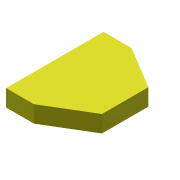
# Autodesk Inventor part: 30_Cube_Z_Focus_Drylin_NEMA_slide_part1
Saved by Autodesk Inventor 2022 (Build 260153000, 153)
## iProperties
Created: 2021-05-05
Part Number: 30_Cube_Z_Focus_Drylin_NEMA_slide_part1
Material: Generic
Document SubType Name: Modeling
Designer: diederichbenedict
Density: 1 g/cm^3
Appearance: Smooth - Yellow
Author: diederichbenedict
Autodesk Inventor part; units mm, degrees
ref_plane "YZ Plane" through (0, 0, 0) normal (1, 0, 0) x (0, 1, 0)
ref_plane "XZ Plane" through (0, 0, 0) normal (0, 1, 0) x (-1, 0, 0)
ref_plane "XY Plane" through (0, 0, 0) normal (0, 0, 1) x (1, 0, 0)
sketch "Sketch1" plane through (0, 0, 0) normal (0, 1, 0) x (-1, 0, 0)
  line L0 (-13, -11.9282) -> (10, -11.9282)
  line L1 (10, -11.9282) -> (10, 11.9282)
  line L2 (10, 11.9282) -> (-13, 11.9282)
  line L3 (-13, 11.9282) -> (-13, -11.9282)
  circle A0 centre (-8, 0) radius 4
  circle A1 centre (4, -6.9282) radius 4
  circle A2 centre (4, 6.9282) radius 4
  circle A3 centre (0, 0) radius 8 construction
  circle A4 centre (0, 0) radius 1.75
  dimension "d11" = 16
  dimension "d2" = 8
  dimension "d6" = 360
  dimension "d8" = 6
  dimension "d9" = 5
  dimension "d12" = 5
  dimension "d13" = 5
  dimension "d35" = 3.5
  constraints: 8 end point, 4 centre point, 3 coincident, 2 parallel, 1 horizontal, 1 horizontal alignment, 1 perpendicular, 9 other
  measures "d2" diameter of A0
  measures "d8" distance from line of A2.centre L1
  measures "d9" distance from line of L3 A0.centre
  measures "d12" distance from line of L2 A2.centre
  measures "d13" distance from line of L0 A1.centre
  measures "d35" diameter of A4
extrude "Extrusion1" add sketch "Sketch1" along normal blind 3
sketch "Sketch2" plane through (0, 3, 0) normal (0, 1, 0) x (1, 0, 0)
  circle A0 centre (-4, -6.9282) radius 4 projected
  circle A1 centre (-4, 6.9282) radius 4 projected
  circle A2 centre (8, 0) radius 4 projected
  line L0 (13, 11.9282) -> (-10, 11.9282) projected
  line L1 (-10, 11.9282) -> (-10, -11.9282) projected
  line L2 (-10, -11.9282) -> (13, -11.9282) projected
  line L3 (13, -11.9282) -> (13, 11.9282) projected
  circle A3 centre (0, 0) radius 1.75
  dimension "d16" = 3.5
  constraints: 1 centre point, 1 coincident
  measures "d16" diameter of A3
extrude "Extrusion2" add sketch "Sketch2" along normal blind 1.5 contours A0 | A1 | A2 | L3 L2 L1 L0
sketch "Sketch3" plane through (0, 0, 0) normal (0, -1, 0) x (1, 0, 0)
  circle A0 centre (-4, 6.9282) radius 4 projected
  circle A1 centre (-4, -6.9282) radius 4 projected
  circle A2 centre (8, 0) radius 4 projected
  line L0 (13, -11.9282) -> (-10, -11.9282) projected
  line L1 (13, 11.9282) -> (13, -11.9282) projected
  line L2 (-10, 11.9282) -> (13, 11.9282) projected
  line L3 (-10, -11.9282) -> (-10, 11.9282) construction
  line L4 (-2, 11.9282) -> (13, 2.9282)
  line L5 (13, 11.9282) -> (13, -11.9282) projected
  line L6 (13, -2.9282) -> (-2, -11.9282)
  point P0 (0, 0)
  dimension "d19" = 9
  dimension "d20" = 9
  dimension "d21" = 15
  dimension "d22" = 15
  constraints: 4 end point, 4 point on line
  measures "d19" distance from line of L2 L4.end
  measures "d20" distance from line of L0 L6.start
  measures "d21" distance from line of L6.end L1
  measures "d22" distance from line of L1 L4.start
extrude "Extrusion3" cut sketch "Sketch3" against normal through all contours L4 L2 L1 | L0 L6 L1
sketch "Sketch5" plane through (0, 0, 0) normal (0, -1, 0) x (1, 0, 0)
  line L0 (13, 2.9282) -> (-2, 11.9282) projected
  line L1 (-10, 11.9282) -> (-2, 11.9282) projected
  line L2 (-10, -11.9282) -> (-10, 11.9282) projected
  line L3 (-2, -11.9282) -> (-10, -11.9282) projected
  line L4 (-2, -11.9282) -> (13, -2.9282) projected
  line L5 (13, 2.9282) -> (13, -2.9282) projected
  circle A0 centre (-4, 6.9282) radius 4 projected
  circle A1 centre (-4, -6.9282) radius 4 projected
  circle A2 centre (8, 0) radius 4 projected
  line L6 (17, -5.193) -> (-0.8921, -15.9282)
  line L7 (-0.8921, -15.9282) -> (-14, -15.9282)
  line L8 (-14, -15.9282) -> (-14, 15.9282)
  line L9 (-14, 15.9282) -> (-0.8921, 15.9282)
  line L10 (-0.8921, 15.9282) -> (17, 5.193)
  line L11 (17, 5.193) -> (17, -5.193)
  line L12 (13, -2.9282) -> (13, -7.593)
  line L13 (13, 2.8448) -> (13, 7.593)
  line L14 (-2, -11.9282) -> (-10, -11.9282) projected
  line L15 (-10, -11.9282) -> (-10, -15.9282)
  line L16 (-10, 11.9282) -> (-2, 11.9282) projected
  line L17 (-10, 11.9282) -> (-10, 15.9282)
  line L18 (-2, -11.9282) -> (13, -2.9282) projected
  line L19 (13, -2.9282) -> (-2, -11.9282)
  line L20 (-2, -11.9282) -> (-10, -11.9282)
  line L21 (-10, -11.9282) -> (-10, 11.9282) projected
  line L22 (-10, 11.9282) -> (-2, 11.9282)
  line L23 (13, 2.9282) -> (-2, 11.9282) projected
  line L24 (13, 2.9282) -> (-2, 11.9282)
  line L25 (13, -2.9282) -> (13, 2.8448)
  point P0 (0, 0)
  dimension "d27" = 4
  constraints: 30 end point, 6 point on line, 4 collinear, 2 perpendicular, 2 vertical, 5 other
  measures "d27" distance between parallel lines of L4 L6
extrude "Extrusion5" add sketch "Sketch5" against normal up to surface (4.5 mm away) contours L0 L1 L17 L9 L10 L13 | L12 L6 L7 L15 L3 L4
sketch "Sketch6" plane through (0, 4.5, 0) normal (0, 1, 0) x (1, 0, 0)
  line L0 (13, -7.593) -> (13, 7.593) projected
  line L1 (-0.8921, 15.9282) -> (13, 7.593) projected
  line L2 (-10, 15.9282) -> (-0.8921, 15.9282) projected
  line L3 (-10, -15.9282) -> (-10, 15.9282) projected
  line L4 (-0.8921, -15.9282) -> (-10, -15.9282) projected
  line L5 (13, -7.593) -> (-0.8921, -15.9282) projected
  line L6 (13, 7.593) -> (-0.8921, 15.9282)
  line L7 (-0.8921, 15.9282) -> (-2.4356, 13.3557)
  line L8 (-2.4356, 13.3557) -> (11.4565, 5.0205)
  line L9 (11.4565, 5.0205) -> (13, 7.593)
  line L10 (13, -7.593) -> (13, 7.593) projected
  line L11 (13, -7.593) -> (-0.8921, -15.9282)
  line L12 (-0.8921, -15.9282) -> (-2.4356, -13.3557)
  line L13 (-2.4356, -13.3557) -> (11.4565, -5.0205)
  line L14 (11.4565, -5.0205) -> (13, -7.593)
  point P0 (0, 0)
  dimension "d30" = 3
  dimension "d31" = 3
  constraints: 16 end point, 5 equal length, 2 perpendicular
  measures "d30" distance of L7.end L1.start
  measures "d31" distance of L4.start L12.end
extrude "Extrusion6" [suppressed]
sketch "Sketch7" plane through (0, 4.5, 0) normal (0, 1, 0) x (1, 0, 0)
  line L0 (13, -7.593) -> (13, 7.593) projected
  line L1 (-0.8921, 15.9282) -> (13, 7.593) projected
  line L2 (-10, 15.9282) -> (-0.8921, 15.9282) projected
  line L3 (-10, -15.9282) -> (-10, 15.9282) projected
  line L4 (-0.8921, -15.9282) -> (-10, -15.9282) projected
  line L5 (13, -7.593) -> (-0.8921, -15.9282) projected
  circle A0 centre (0, 0) radius 1.75 projected
  line L6 (1.6166, 2.8) -> (3.2332, 0)
  line L7 (3.2332, 0) -> (1.6166, -2.8)
  line L8 (1.6166, -2.8) -> (-1.6166, -2.8)
  line L9 (-1.6166, -2.8) -> (-3.2332, 0)
  line L10 (-3.2332, 0) -> (-1.6166, 2.8)
  line L11 (-1.6166, 2.8) -> (1.6166, 2.8)
  line L12 (-1.6166, 2.8) -> (-11.6048, 2.8)
  line L13 (-11.6048, 2.8) -> (-11.6048, -2.8)
  line L14 (-11.6048, -2.8) -> (-1.6166, -2.8)
  line L15 (-1.6166, -2.8) -> (-1.6166, 2.8)
  dimension "d39" = 5.6
  constraints: 20 end point, 3 parallel, 1 coincident, 1 horizontal, 1 perpendicular, 13 other
  measures "d39" distance between parallel lines of L8 L11
extrude "Extrusion7" cut sketch "Sketch7" against normal blind 3.5 contours L14 L13 L12 L3 | L3 L12 L10 L9 L14 | L15 A0 L11 L6 L7 L8 | L9 L10 L15 A0
sketch "Sketch8" plane through (0, 4.5, 0) normal (0, 1, 0) x (1, 0, 0)
  line L0 (-10, 2.8) -> (1.6166, 2.8) projected
  line L1 (1.6166, 2.8) -> (3.2332, 0) projected
  line L2 (3.2332, 0) -> (1.6166, -2.8) projected
  line L3 (1.6166, -2.8) -> (-10, -2.8) projected
  line L4 (-10, -15.9282) -> (-10, -2.8) projected
  line L5 (-0.8921, -15.9282) -> (-10, -15.9282) projected
  line L6 (13, -7.593) -> (-0.8921, -15.9282) projected
  line L7 (13, -7.593) -> (13, 7.593) projected
  line L8 (-0.8921, 15.9282) -> (13, 7.593) projected
  line L9 (-10, 15.9282) -> (-0.8921, 15.9282) projected
  line L10 (-10, 2.8) -> (-10, 15.9282) projected
  line L11 (-10, 2.8) -> (-10, 15.9282) projected
  line L12 (-10, -15.9282) -> (-10, -2.8) projected
  line L13 (-10, 2.8) -> (-10, -2.8)
  circle A0 centre (0, 0) radius 1.75 projected
  constraints: 2 end point, 1 collinear
extrude "Extrusion8" add sketch "Sketch8" along normal blind 1
equation "\"d12\" = d9"
equation "\"d13\" = d9"
body "Solid1"
